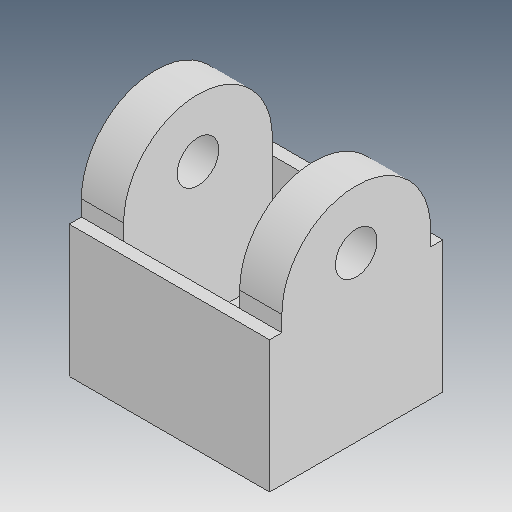
# Autodesk Inventor part: pulley_base
Saved by Autodesk Inventor 2025.2 (Build 292293000, 293)
## iProperties
Created: 2025-02-16
Part Number: pulley_base
Material: Generic
Document SubType Name: Modeling
Designer: email
Density: 1 g/cm^3
Appearance: Default
Author: email
Autodesk Inventor part; units mm, degrees
ref_plane "YZ Plane" through (0, 0, 0) normal (1, 0, 0) x (0, 1, 0)
ref_plane "XZ Plane" through (0, 0, 0) normal (0, 1, 0) x (-1, 0, 0)
ref_plane "XY Plane" through (0, 0, 0) normal (0, 0, 1) x (1, 0, 0)
sketch "Sketch1" plane through (0, 0, 0) normal (0, 0, 1) x (1, 0, 0)
  line L0 (-19, 0) -> (19, 0)
  line L1 (19, 0) -> (19, 42.1)
  line L2 (19, 42.1) -> (11, 42.1)
  line L3 (11, 42.1) -> (11, 5)
  line L4 (11, 5) -> (-11, 5)
  line L5 (-11, 5) -> (-11, 42.1)
  line L6 (-11, 42.1) -> (-19, 42.1)
  line L7 (-19, 42.1) -> (-19, 0)
  point P0 (0, 0)
  dimension "d0" = 22
  dimension "d1" = 5
  dimension "d2" = 37.1
  dimension "d14" = 8
  dimension "d15" = 8
  dimension "d26" = 47.0273
  constraints: 16 end point, 5 perpendicular, 2 midpoint, 2 point on line, 1 horizontal, 1 parallel
  measures "d0" distance between parallel lines of L3 L5
  measures "d1" distance between parallel lines of L0 L4
  measures "d2" distance between parallel lines of L4 L6
  measures "d14" distance between parallel lines of L5 L7
  measures "d15" distance between parallel lines of L1 L3
extrude "Extrusion1" add sketch "Sketch1" along normal blind 28.2
sketch "Sketch2" plane through (-11, 5, 0) normal (0, 1, 0) x (1, 0, 0)
  circle A0 centre (11, -14.1) radius 4.75
  line L0 (22, 0) -> (0, 0) projected
  line L1 (-8, 0) -> (-8, -28.2) projected
  point P0 (11, 0)
  point P1 (11, 0)
  point P2 (-8, -14.1)
  dimension "d6" = 9.5
  constraints: 2 midpoint, 1 centre point, 1 horizontal alignment, 1 vertical alignment
  measures "d6" diameter of A0
extrude "Extrusion2" cut sketch "Sketch2" against normal up to next
sketch "Sketch3" plane through (19, 0, 0) normal (1, 0, 0) x (0, 0, -1)
  line L0 (0, 5) -> (-28.2, 5) projected
  circle A0 centre (-14.1, 31.05) radius 3.95
  line L1 (0, 0) -> (0, 42.1) projected
  line L2 (0, 42.1) -> (-28.2, 42.1) projected
  point P0 (-14.1, 42.1)
  dimension "d9" = 7.9
  dimension "d11" = 26.05
  constraints: 1 centre point, 1 midpoint, 1 vertical alignment
  measures "d9" diameter of A0
  measures "d11" distance from line of L0 A0.centre
extrude "Extrusion3" cut sketch "Sketch3" against normal through all
sketch "Sketch4" plane through (19, 0, 0) normal (1, 0, 0) x (0, 0, -1)
  line L0 (-28.2, 0) -> (-28.2, 42.1) projected
  line L1 (-28.2, 27.157) -> (-28.2, 0)
  circle A0 centre (-14.1, 31.05) radius 17.5
  circle A1 centre (-14.1, 31.05) radius 14.1
  line L2 (-28.2, 0) -> (-30.5209, 0)
  line L3 (-30.5209, 0) -> (-30.5209, 25)
  line L4 (-30.5209, 25) -> (-28.2, 25)
  line L5 (-28.2, 25) -> (-28.2, 0)
  line L6 (0, 0) -> (2.3209, 0)
  line L7 (2.3209, 0) -> (2.3209, 25)
  line L8 (2.3209, 25) -> (0, 25)
  line L9 (0, 25) -> (0, 0)
  dimension "d23" = 35
  dimension "d24" = 28.2
  dimension "d25" = 25
  constraints: 18 end point, 4 parallel, 2 centre point, 2 coincident, 2 horizontal, 2 perpendicular, 2 point on circle, 1 point on line
  measures "d23" diameter of A0
  measures "d24" diameter of A1
  measures "d25" distance of L2.end L3.end
extrude "Extrusion4" add sketch "Sketch4" against normal up to surface (38 mm away) contours L0 A0 L4 | L0 L2 L3 A0 | L9 L8 A0 | A0 L7 L6 L9 picked at (-28.5025, 22.5777)
full round fillet "Full Round Fillet1" first side at (-13.6667, 36.4, 28.2) centre faces at (-13.6667, 42.1, 9.4) second side at (-13.6667, 36.4, 0)
full round fillet "Full Round Fillet2" first side at (13.6667, 36.4, 28.2) centre faces at (16.3333, 42.1, 9.4) second side at (13.6667, 36.4, 0)
body "Solid1"
